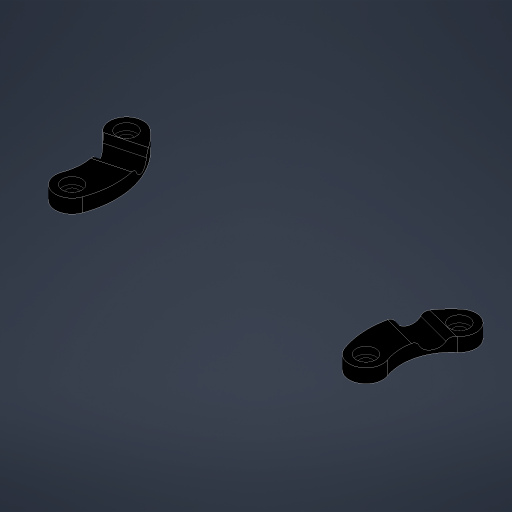
# Autodesk Inventor part: MettalringUnten_v3
Saved by Autodesk Inventor 2023.2 (Build 272271030, 271C)
## iProperties
Created: 2022-10-10
Part Number: MettalringUnten_v3
Material: Generic
Document SubType Name: Modeling
Designer: braun
Density: 1 g/cm^3
Appearance: Default
Author: braun
Autodesk Inventor part; units mm, degrees
ref_plane "YZ Plane" through (0, 0, 0) normal (1, 0, 0) x (0, 1, 0)
ref_plane "XZ Plane" through (0, 0, 0) normal (0, 1, 0) x (-1, 0, 0)
ref_plane "XY Plane" through (0, 0, 0) normal (0, 0, 1) x (1, 0, 0)
sketch "Sketch1" plane through (0, 0, 0) normal (0, 1, 0) x (-1, 0, 0)
  circle A0 centre (0, 0) radius 110 construction
  arc A1 (43.0581, -98.5) -> (-43.0581, -98.5) centre (0, 0) ccw
  line L0 (0, -107.5) -> (0, -98.5) construction
  line L1 (0, -98.5) -> (0, -73.5) construction
  line L2 (0, -98.5) -> (-43.0581, -98.5) construction
  line L3 (0, -98.5) -> (43.0581, -98.5) construction
  line L4 (43.0581, -98.5) -> (-43.0581, -98.5) construction
  line L5 (-18.0581, -73.5) -> (18.0581, -73.5)
  arc A2 (43.0581, -98.5) -> (18.0581, -73.5) centre (18.0581, -98.5) ccw
  arc A3 (-18.0581, -73.5) -> (-43.0581, -98.5) centre (-18.0581, -98.5) ccw
  line L6 (0, 107.5) -> (0, 97.5) construction
  line L7 (0, 97.5) -> (-22.5, 97.5) construction
  line L8 (-22.5, 97.5) -> (-22.5, 82.5) construction
  line L9 (22.5, 82.5) -> (22.5, 97.5) construction
  line L10 (22.5, 90) -> (-22.5, 90) construction
  line L11 (15, 97.5) -> (-15, 97.5)
  line L12 (-15, 82.5) -> (15, 82.5)
  arc A4 (15, 82.5) -> (15, 97.5) centre (15, 90) ccw
  arc A5 (-15, 97.5) -> (-15, 82.5) centre (-15, 90) ccw
  line L13 (22.5, 82.5) -> (17.5, 82.5) construction
  line L14 (17.5, 82.5) -> (17.5, 77.5) construction
  circle A6 centre (17.5, 77.5) radius 1.6
  circle A7 centre (-17.5, 77.5) radius 1.6
  line L15 (-58.3363, 79.5495) -> (-79.5495, 58.3363)
  arc A8 (-47.7297, 68.9429) -> (-58.3363, 79.5495) centre (-53.033, 74.2462) ccw
  arc A9 (-79.5495, 58.3363) -> (-68.9429, 47.7297) centre (-74.2462, 53.033) ccw
  line L16 (-68.9429, 47.7297) -> (-47.7297, 68.9429)
  circle A10 centre (-67.1751, 42.4264) radius 1.6
  circle A11 centre (-42.4264, 67.1751) radius 1.6
  line L17 (-97.5, 15) -> (-97.5, -15)
  arc A12 (-82.5, 15) -> (-97.5, 15) centre (-90, 15) ccw
  arc A13 (-97.5, -15) -> (-82.5, -15) centre (-90, -15) ccw
  line L18 (-82.5, -15) -> (-82.5, 15)
  circle A14 centre (-77.5, -17.5) radius 1.6
  circle A15 centre (-77.5, 17.5) radius 1.6
  line L19 (-79.5495, -58.3363) -> (-58.3363, -79.5495)
  arc A16 (-68.9429, -47.7297) -> (-79.5495, -58.3363) centre (-74.2462, -53.033) ccw
  arc A17 (-58.3363, -79.5495) -> (-47.7297, -68.9429) centre (-53.033, -74.2462) ccw
  line L20 (-47.7297, -68.9429) -> (-68.9429, -47.7297)
  circle A18 centre (-42.4264, -67.1751) radius 1.6
  circle A19 centre (-67.1751, -42.4264) radius 1.6
  line L21 (-15, -97.5) -> (15, -97.5)
  arc A20 (-15, -82.5) -> (-15, -97.5) centre (-15, -90) ccw
  arc A21 (15, -97.5) -> (15, -82.5) centre (15, -90) ccw
  line L22 (15, -82.5) -> (-15, -82.5)
  circle A22 centre (17.5, -77.5) radius 1.6
  circle A23 centre (-17.5, -77.5) radius 1.6
  line L23 (58.3363, -79.5495) -> (79.5495, -58.3363)
  arc A24 (47.7297, -68.9429) -> (58.3363, -79.5495) centre (53.033, -74.2462) ccw
  arc A25 (79.5495, -58.3363) -> (68.9429, -47.7297) centre (74.2462, -53.033) ccw
  line L24 (68.9429, -47.7297) -> (47.7297, -68.9429)
  circle A26 centre (67.1751, -42.4264) radius 1.6
  circle A27 centre (42.4264, -67.1751) radius 1.6
  line L25 (97.5, -15) -> (97.5, 15)
  arc A28 (82.5, -15) -> (97.5, -15) centre (90, -15) ccw
  arc A29 (97.5, 15) -> (82.5, 15) centre (90, 15) ccw
  line L26 (82.5, 15) -> (82.5, -15)
  circle A30 centre (77.5, 17.5) radius 1.6
  circle A31 centre (77.5, -17.5) radius 1.6
  line L27 (79.5495, 58.3363) -> (58.3363, 79.5495)
  arc A32 (68.9429, 47.7297) -> (79.5495, 58.3363) centre (74.2462, 53.033) ccw
  arc A33 (58.3363, 79.5495) -> (47.7297, 68.9429) centre (53.033, 74.2462) ccw
  line L28 (47.7297, 68.9429) -> (68.9429, 47.7297)
  circle A34 centre (42.4264, 67.1751) radius 1.6
  circle A35 centre (67.1751, 42.4264) radius 1.6
  line L29 (58.3363, -58.3363) -> (51.2652, -51.2652) construction
  line L30 (40.6586, -61.8718) -> (61.8718, -40.6586)
  arc A36 (40.6586, -61.8718) -> (44.5267, -89.5398) centre (53.033, -74.2462) ccw
  arc A37 (89.5398, -44.5267) -> (61.8718, -40.6586) centre (74.2462, -53.033) ccw
  line L31 (0, -73.5) -> (0, -66.5) construction
  arc A38 (44.5267, 89.5398) -> (40.6586, 61.8718) centre (53.033, 74.2462) ccw
  line L32 (61.8718, 40.6586) -> (40.6586, 61.8718)
  arc A39 (61.8718, 40.6586) -> (89.5398, 44.5267) centre (74.2462, 53.033) ccw
  arc A40 (-89.5398, 44.5267) -> (-61.8718, 40.6586) centre (-74.2462, 53.033) ccw
  line L33 (-40.6586, 61.8718) -> (-61.8718, 40.6586)
  arc A41 (-40.6586, 61.8718) -> (-44.5267, 89.5398) centre (-53.033, 74.2462) ccw
  arc A42 (-44.5267, -89.5398) -> (-40.6586, -61.8718) centre (-53.033, -74.2462) ccw
  line L34 (-61.8718, -40.6586) -> (-40.6586, -61.8718)
  arc A43 (-61.8718, -40.6586) -> (-89.5398, -44.5267) centre (-74.2462, -53.033) ccw
  arc A44 (89.5398, -44.5267) -> (89.5398, 44.5267) centre (0, 0) ccw
  arc A45 (44.5267, 89.5398) -> (-44.5267, 89.5398) centre (0, 0) ccw
  arc A46 (-89.5398, 44.5267) -> (-89.5398, -44.5267) centre (0, 0) ccw
  line L35 (43.0581, -98.5) -> (48.0581, -98.5) construction
  line L36 (48.0581, -98.5) -> (48.0581, -88.5) construction
  circle A47 centre (48.0581, -88.5) radius 1.6
  circle A48 centre (-48.0581, -88.5) radius 1.6
  line L37 (18.0581, -66.5) -> (-18.0581, -66.5)
  arc A49 (17.5, -66.5) -> (43.0581, -59.4724) centre (19.5145, -23.8377) ccw
  arc A50 (-44.5267, -58.0038) -> (-18.0581, -66.5) centre (-19.5089, -25.5422) ccw
  arc A51 (-48.0581, -88.5) -> (-42.4264, -67.1751) centre (-60.4397, -73.8241) ccw construction
  arc A52 (-48.0581, -88.5) -> (-42.4264, -67.1751) centre (-60.4397, -73.8241) ccw construction
  arc A53 (-44.9367, -92.1998) -> (-37.8853, -65.499) centre (-60.4397, -73.8241) ccw
  arc A54 (-51.1795, -84.8002) -> (-46.9675, -68.8513) centre (-60.4397, -73.8241) ccw
  arc A55 (-51.1795, -84.8002) -> (-44.9367, -92.1998) centre (-48.0581, -88.5) ccw
  arc A56 (-37.8853, -65.499) -> (-46.9675, -68.8513) centre (-42.4264, -67.1751) ccw
  point P0 (0, 90)
  point P1 (-45.9619, 70.7107)
  point P2 (-82.5, 17.5)
  point P3 (-70.7107, -45.9619)
  point P4 (-17.5, -82.5)
  point P5 (45.9619, -70.7107)
  point P6 (82.5, -17.5)
  point P7 (70.7107, 45.9619)
  point P8 (35.7159, -76.7698)
  point P9 (-37.9023, -65.4535)
  point P10 (-39.0971, -63.6613)
  point P11 (-46.4221, -70.7043)
  point P12 (-46.8673, -78.5164)
  point P13 (0, -44.5267)
  point P14 (0, 35.7016)
  dimension "d0" = 220
  dimension "d1" = 215
  dimension "d2" = 9
  dimension "d3" = 25
  dimension "d4" = 10
  dimension "d5" = 22.5
  dimension "d6" = 15
  dimension "d7" = 45
  dimension "d8" = 5
  dimension "d9" = 5
  dimension "d10" = 3.2
  dimension "d15" = 86.1162
  dimension "d16" = 45
  dimension "d19" = 360
  dimension "d22" = 10
  dimension "d23" = 7
  dimension "d26" = 360
  dimension "d33" = 5
  dimension "d34" = 10
  dimension "d35" = 3.2
  constraints: 82 point on circle, 80 end point, 57 centre point, 19 point on line, 12 tangent, 5 coincident, 5 midpoint, 4 vertical, 2 horizontal, 2 symmetric about line, 1 collinear, 1 parallel, 1 perpendicular, 160 other
  measures "d0" diameter of A0
  measures "d1" diameter of A1
  measures "d2" distance of L0.start L0.end
  measures "d3" distance of L0.end L1.end
  measures "d4" distance of L6.start L6.end
  measures "d5" distance of L6.end L7.end
  measures "d6" distance of L7.end L8.end
  measures "d7" distance of L8.end L9.start
  measures "d8" distance of L9.start L13.end
  measures "d9" distance of L13.end L14.end
  measures "d10" diameter of A6
  measures "d15" distance of L3.end L2.end
  measures "d16" distance of L10.start L10.end
  measures "d22" distance of L29.start L29.end
  measures "d23" distance of L1.end L31.end
  measures "d33" distance of L3.end L35.end
  measures "d34" distance of L35.end L36.end
  measures "d35" diameter of A47
extrude "Extrusion5" add sketch "Sketch1" along normal blind 4 contours A53 A55 A54 A17 A56 A42 | A42 A56 | A54 A17
sketch "Sketch6" plane through (0, 4, 0) normal (0, 1, 0) x (1, 0, 0)
  circle A0 centre (42.4264, 67.1751) radius 1.6 projected
  circle A1 centre (42.4264, 67.1751) radius 2.8
  circle A2 centre (48.0581, 88.5) radius 1.6 projected
  circle A3 centre (48.0581, 88.5) radius 2.8
  point P0 (0, 0)
  dimension "d56" = 5.6
  dimension "d57" = 5.6
  constraints: 2 centre point, 2 coincident
  measures "d56" diameter of A1
  measures "d57" diameter of A3
extrude "Extrusion6" cut sketch "Sketch6" against normal blind 2 contours A0 | A1 | A2 | A3
ref_plane "Work Plane2" through (37.8853, 0, -65.499) normal (-0.9668522, 0, -0.2553366) x (0, 1, 0)
sketch "Sketch7" plane through (37.8853, 0, -65.499) normal (-0.9668522, 0, -0.2553366) x (0, 1, 0)
  line L0 (0, 27.6163) -> (4, 27.6163) projected
  line L1 (2, 27.6163) -> (2, 0) construction
  line L2 (0, 0) -> (4, 0) projected
  line L3 (2, 13.8081) -> (5.6788, 13.8081) construction
  line L4 (5.6788, 13.8081) -> (5.6788, 17.3081) construction
  line L5 (5.6788, 17.3081) -> (4, 17.3081) construction
  line L6 (4, 0) -> (4, 27.6163) construction
  circle A0 centre (4, 17.3081) radius 3
  point P0 (0, -73.0013)
  dimension "d60" = 27.6163
  dimension "d61" = 13.8081
  dimension "d62" = 3.5
  dimension "d63" = 6
  constraints: 8 end point, 2 midpoint, 1 centre point, 1 coincident, 1 perpendicular, 1 point on line, 1 vertical
  measures "d60" distance of L1.start L1.end
  measures "d61" distance of point (2, 27.616) L3.start
  measures "d62" distance of L3.end L4.end
  measures "d63" diameter of A0
extrude "Extrusion7" cut sketch "Sketch7" along normal mid plane 19.75
fillet "Fillet3" radius 2 2 edges at (44.7193, 4, -84.6985) (42.0093, 4, -79.2085)
sketch "Sketch8" plane through (0, 4, 0) normal (0, 1, 0) x (1, 0, 0)
  point P0 (0, 0)
  point P1 (0, 45.0877)
  point P2 (0, -47.4612)
ref_plane "Work Plane4" through (0, 0, -44.5267) normal (1, 0, 0) x (0, 0.9903099, -0.1388753)
mirror "Mirror2" about plane through (0, 0, -44.5267) normal (1, 0, 0) of "Extrusion5", "Extrusion6", "Extrusion7", "Fillet3"
ref_plane "Work Plane5" through (-37.8853, 0, -65.499) normal (-0.9668522, 0, 0.2553366) x (0, 1, 0)
body "Solid2"
